Autodesk Fusion 360 part; units mm, degrees
(part 2 of 2)
sketch "Sketch3" plane through (0, -51, 0) normal (0, -1, 0) x (1, 0, 0)
  line L0 (-36, 0) -> (36, 0)
  line L1 (36, 0) -> (36, 24.7)
  line L2 (36, 24.7) -> (-36, 24.7)
  line L3 (-36, 24.7) -> (-36, 0)
  line L4 (-26.5, 21.7) -> (-10.5, 21.7)
  line L5 (-10.5, 21.7) -> (-10.5, 4.7)
  line L6 (-10.5, 4.7) -> (-26.5, 4.7)
  line L7 (-26.5, 4.7) -> (-26.5, 21.7)
  circle A0 centre (16, 11) radius 1.5
  circle A1 centre (25, 13.7) radius 3
  line L8 (-18.5, 21.7) -> (-18.5, 4.7) construction
  line L9 (-26.5, 13.2) -> (-10.5, 13.2) construction
  line L10 (-25, 18.8) -> (-12, 18.8)
  line L11 (-12, 18.8) -> (-12, 7.9)
  line L12 (-12, 7.9) -> (-25, 7.9)
  line L13 (-25, 7.9) -> (-25, 18.8)
  line L14 (-15.25, 7.9) -> (-21.75, 7.9)
  line L15 (-21.75, 7.9) -> (-21.75, 6)
  line L16 (-21.75, 6) -> (-15.25, 6)
  line L17 (-15.25, 6) -> (-15.25, 7.9)
  line L18 (-15.25, 7.9) -> (-21.75, 6) construction
  line L19 (-21.75, 7.9) -> (-15.25, 6) construction
  line L20 (6, 18.8) -> (6, 7.9)
  line L21 (7.5, 21.7) -> (7.5, 4.7)
  line L22 (-7, 7.9) -> (-7, 18.8)
  line L23 (-8.5, 21.7) -> (7.5, 21.7)
  line L24 (-3.75, 7.9) -> (2.75, 6) construction
  line L25 (6, 7.9) -> (-7, 7.9)
  line L26 (-3.75, 7.9) -> (-3.75, 6)
  line L27 (-7, 18.8) -> (6, 18.8)
  line L28 (-8.5, 4.7) -> (-8.5, 21.7)
  line L29 (-8.5, 13.2) -> (7.5, 13.2) construction
  line L30 (-3.75, 6) -> (2.75, 6)
  line L31 (2.75, 6) -> (2.75, 7.9)
  line L32 (2.75, 7.9) -> (-3.75, 6) construction
  line L33 (-0.5, 21.7) -> (-0.5, 4.7) construction
  line L34 (2.75, 7.9) -> (-3.75, 7.9)
  line L35 (7.5, 4.7) -> (-8.5, 4.7)
  circle A2 centre (25, 13.7) radius 0.7
  line L36 (-36, 0) -> (36, 0)
  line L37 (20.725, 18) -> (29.275, 18)
  line L38 (29.275, 18) -> (29.275, 7)
  line L39 (29.275, 7) -> (20.725, 7)
  line L40 (20.725, 7) -> (20.725, 18)
  line L41 (25, 13.7) -> (25, 18) construction
  point P0 (-18.5, 6.95)
  point P1 (-0.5, 6.95)
  dimension "d44" = 16
  dimension "d45" = 17
  dimension "d46" = 1.5
  dimension "d47" = 1.5
  dimension "d48" = 2.9
  dimension "d49" = 3.2
  dimension "d50" = 1.3
  dimension "d51" = 6.5
  dimension "d52" = 9.5
  dimension "d53" = 3
  dimension "d56" = 18
  dimension "d57" = 0
  dimension "d58" = 3
  dimension "d59" = 6
  dimension "d60" = 1.4
  dimension "d61" = 11
  dimension "d62" = 11
  dimension "d63" = 11
  dimension "d64" = 20
  dimension "d67" = 11
  dimension "d68" = 4.3
  dimension "d69" = 8.55
  constraint horizontal L4
  constraint vertical L5
  constraint horizontal L6
  constraint vertical L7
  constraint midpoint L4 L8.start
  constraint midpoint L6 L8.end
  constraint midpoint L7 L9.start
  constraint midpoint L5 L9.end
  constraint horizontal L10
  constraint vertical L11
  constraint horizontal L12
  constraint vertical L13
  constraint horizontal L14
  constraint perpendicular L14 L15
  constraint parallel L14 L16
  constraint parallel L15 L17
  constraint coincident L12 L14.start
  constraint coincident L18 P0
  constraint coincident L19 P0
  constraint coincident L8 P0
  constraint concentric A1 A2
  constraint horizontal L37
  constraint vertical L38
  constraint horizontal L39
  constraint vertical L40
  constraint coincident A1.centre A2.centre
  constraint vertical L41
  constraint symmetric L38 L40 L41
  measures "d44" distance of L5 L7
  measures "d45" distance of L4 L6
  measures "d46" distance of L5 L11
  measures "d47" distance of L7 L13
  measures "d48" distance of L4 L10
  measures "d49" distance of L6 L12
  measures "d50" distance of L6 L16
  measures "d51" distance of L15 L17
  measures "d52" distance of L3 L7
  measures "d53" distance of L2 L4
  measures "d58" diameter of A0
  measures "d59" diameter of A1
  measures "d60" diameter of A2
  measures "d61" distance of L1 A1.centre
  measures "d62" distance of L2 A1.centre
  measures "d63" distance of A0.centre L36
  measures "d64" distance of L1 A0.centre
  measures "d67" distance of L37 L39
  measures "d68" distance of A1.centre L37
  measures "d69" distance of L38 L40
extrude "Extrude5" add sketch "Sketch3" along normal blind 0.3 separate body contours L4 L5 L6 L7 | L21 L23 L28 L35 | L37 L38 L39 L40 makes body 13 at (-2.6667, -51, 20.7333) makes body 14 at (-16.3333, -51, 20.7333) makes body 15 at (24.9253, -51, 8.2361)
extrude "Extrude6" cut sketch "Sketch3" against normal blind 9.6 contours A1 | L10 L11 L12 L13 L14 | L12 L14 L15 L16 L17 | L20 L22 L25 L27 L34 | L25 L26 L30 L31 L34 bodies 1 15 14 13 12 11 10 3 4 9 8 7 6 5 2
extrude "Extrude7" cut sketch "Sketch3" against normal blind 3 contours A0 bodies 11 6 14 13 4 5 10 2 15 3 1 7 12 8 9
sketch "Sketch4" plane through (-36, 0, 0) normal (-1, 0, 0) x (0, -1, 0)
  line L0 (12.6, 1) -> (12.6, 0)
  line L1 (12.6, 0) -> (51, 0)
  line L2 (51, 0) -> (51, 24.7)
  line L3 (51, 24.7) -> (-51, 24.7)
  line L4 (-51, 24.7) -> (-51, 0)
  line L5 (-51, 0) -> (-13.7, 0)
  line L6 (-13.7, 0) -> (-13.7, 1)
  line L7 (-13.7, 1) -> (12.6, 1)
  line L8 (-44, 24.7) -> (-25, 24.7)
  line L9 (-25, 24.7) -> (-25, 0)
  line L10 (-25, 0) -> (-44, 0)
  line L11 (-44, 0) -> (-44, 24.7)
  line L12 (-40.5282, 9.0263) -> (-24.62, 9.0263) construction
  line L13 (-24.62, 9.0263) -> (-24.62, 20.5347) construction
  line L14 (-24.62, 20.5347) -> (-40.5282, 20.5347) construction
  line L15 (-40.5282, 20.5347) -> (-40.5282, 9.0263) construction
  dimension "d74" = 19
  dimension "d75" = 7
  dimension "d78" = 5
  text T0 "SIM" font "Arial" height 5 align left top in box 15.9082 x 11.5083 at (-40.5282, 9.0263) x (1, 0) y (0, 1) spacing 1 kerned
  constraint horizontal L8
  constraint vertical L9
  constraint horizontal L10
  constraint vertical L11
  constraint coincident L3 L8.start
  constraint collinear L5 L10
  measures "d74" distance of L9 L11
  measures "d75" distance of L4 L11
extrude "Extrude8" cut sketch "Sketch4" against normal blind 0.2 contours L3 L5 L8 L9 L10 L11 bodies 9 3 8 13 14 6 7 2 4 1 11 12 10 15 5
extrude "Extrude9" cut sketch "Sketch4" against normal blind 2 text T0 bodies 10 13 1 15 3 12 4 14 9 7 2 8 11 5 6
fillet "Fillet1" radius 1 11 edges at (0, -51, 24.7) (36, 0, 24.7) (36, -51, 12.35) (-36, -13, 24.7) (-36, -51, 12.35) (36, 51, 12.35) (0, 51, 24.7) (-36, 47.5, 24.7) (-35.8, 34.5, 24.7) (-36, 51, 12.35) (-36, 0.55, 1) on bodies 1
equation "d3 = ( 96.2 / 2 ) * 1 mm"
equation "d6 = 16.8 mm - d5"
equation "d7 = 2.45 mm + ( d5 / 2 )"
equation "d9 = 4 mm + d5 / 2"
equation "d11 = 2.2 mm + d10 / 2"
equation "d17 = ( 8 / 2 ) * 1 mm"
equation "d47 = d46"

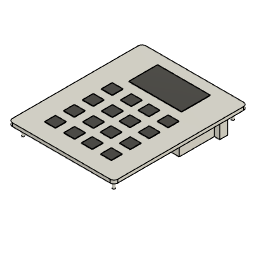
design "CD-100"
Autodesk Fusion 360 part; units mm, degrees
sketch "Cutout" plane through (0, 0, 0) normal (0, 0, 1) x (1, 0, 0)
  line L0 (68.7, -87) -> (-68.7, -87)
  line L1 (-68.7, -87) -> (-68.7, 87)
  line L2 (-68.7, 87) -> (68.7, 87)
  line L3 (68.7, 87) -> (68.7, -87)
  line L4 (68.7, -87) -> (-68.7, 87) construction
  line L5 (-68.7, -87) -> (68.7, 87) construction
  circle A0 centre (-59.055, 77.6351) radius 1.905
  line L6 (0, 0) -> (0, 100) construction
  circle A1 centre (59.055, 77.6351) radius 1.905
  line L7 (0, 0) -> (90, 0) construction
  circle A2 centre (59.055, -77.6351) radius 1.905
  circle A3 centre (-59.055, -77.6351) radius 1.905
  line L8 (-52.9971, 77.6351) -> (52.9971, 77.6351)
  line L9 (52.9971, 77.6351) -> (52.9971, 6.5913)
  line L10 (52.9971, 6.5913) -> (-52.9971, 6.5913)
  line L11 (-52.9971, 6.5913) -> (-52.9971, 77.6351)
  line L12 (-59.055, 72.4281) -> (59.055, 72.4281)
  line L13 (59.055, 72.4281) -> (59.055, 59.7281)
  line L14 (59.055, 59.7281) -> (-59.055, 59.7281)
  line L15 (-59.055, 59.7281) -> (-59.055, 72.4281)
  dimension "d1" = 137.4
  dimension "d2" = 174
  dimension "d7" = 3.81
  dimension "d10" = 118.11
  dimension "d11" = 155.2702
  dimension "d12" = 105.9942
  dimension "d13" = 71.0438
  dimension "d14" = 5.207
  dimension "d15" = 118.11
  dimension "d16" = 12.7
  constraint horizontal L0
  constraint perpendicular L0 L1
  constraint parallel L0 L2
  constraint parallel L1 L3
  constraint coincident L4 L6.start
  constraint coincident L5 L6.start
  constraint coincident L6.start L7.start
  constraint vertical L6
  constraint symmetric A0 L6 A1
  constraint perpendicular L6 L7
  constraint symmetric A0 L7 A3
  constraint symmetric A1 L7 A2
  constraint horizontal L8
  constraint vertical L9
  constraint horizontal L10
  constraint vertical L11
  constraint symmetric L6 L9 L11
  constraint coincident A0.centre L8
  constraint horizontal L12
  constraint vertical L13
  constraint horizontal L14
  constraint vertical L15
  constraint symmetric L6 L13 L15
  measures "d1" distance of L1.end L2.end
  measures "d2" distance of L0.end L1.end
  measures "d7" diameter of A0
  measures "d10" distance of A0.centre A1.centre
  measures "d11" distance of A0.centre A3.centre
  measures "d12" distance of L9 L11
  measures "d13" distance of L8 L10
  measures "d14" distance of A0.centre L12
  measures "d15" distance of L13 L15
  measures "d16" distance of L12 L14
extrude "Extrude1" add sketch "Cutout" along normal blind 4.3 contours L0 L1 L2 L3 | A0 | A1 | A2 | A3 | L8 L9 L11 L12 | L9 L11 L12 L14 | L11 L12 L14 L15 | L9 L12 L13 L14 | L9 L10 L11 L14 makes body 1
sketch "Sketch2" plane through (0, 0, 4.3) normal (0, 0, 1) x (-1, 0, 0)
  line L0 (-68.7, -87) -> (68.7, -87)
  line L1 (68.7, -87) -> (68.7, 87)
  line L2 (68.7, 87) -> (-68.7, 87)
  line L3 (-68.7, 87) -> (-68.7, -87)
sketch "Sketch3" plane through (0, 0, 0) normal (0, 0, -1) x (1, 0, 0)
  line L0 (-68.7, -87) -> (68.7, -87)
  line L1 (68.7, -87) -> (68.7, 87)
  line L2 (68.7, 87) -> (-68.7, 87)
  line L3 (-68.7, 87) -> (-68.7, -87)
  line L4 (-51.9, -14.9) -> (51.9, -14.9)
  line L5 (51.9, -14.9) -> (51.9, -76.4)
  line L6 (51.9, -76.4) -> (-51.9, -76.4)
  line L7 (-51.9, -76.4) -> (-51.9, -14.9)
  line L8 (0, 0) -> (0, 115) construction
  line L9 (-68.7, -87) -> (68.7, -87) construction
  line L10 (58.9, -71.1) -> (-58.9, -71.1)
  line L11 (-58.9, -71.1) -> (-58.9, -60.72)
  line L12 (-58.9, -60.72) -> (58.9, -60.72)
  line L13 (58.9, -60.72) -> (58.9, -71.1)
  circle A0 centre (-59.055, 77.6351) radius 1.65
  circle A1 centre (59.055, 77.6351) radius 1.65
  circle A2 centre (59.055, -77.6351) radius 1.65
  circle A3 centre (-59.055, -77.6351) radius 1.65
  point P0 (-59.055, 77.6351)
  point P1 (59.055, 77.6351)
  point P2 (59.055, -77.6351)
  point P3 (-59.055, -77.6351)
  dimension "d17" = 103.8
  dimension "d18" = 61.5
  dimension "d20" = 10.6
  dimension "d21" = 10.38
  dimension "d22" = 15.9
  dimension "d23" = 7
  dimension "d24" = 7
  dimension "d27" = 3.3
  dimension "d28" = 3.3
  dimension "d29" = 3.3
  dimension "d30" = 3.3
  constraint horizontal L4
  constraint vertical L5
  constraint horizontal L6
  constraint vertical L7
  constraint coincident L8.start origin
  constraint perpendicular L6 L8
  constraint symmetric L5 L7 L8
  constraint horizontal L10
  constraint vertical L11
  constraint horizontal L12
  constraint vertical L13
  constraint coincident P0 A0.centre
  constraint coincident P1 A1.centre
  constraint coincident P2 A2.centre
  constraint coincident P3 A3.centre
  measures "d17" distance of L5 L7
  measures "d18" distance of L4 L6
  measures "d20" distance of L6 L9
  measures "d21" distance of L10 L12
  measures "d22" distance of L9 L10
  measures "d23" distance of L7 L11
  measures "d24" distance of L5 L13
  measures "d27" diameter of A0
  measures "d28" diameter of A1
  measures "d29" diameter of A2
  measures "d30" diameter of A3
extrude "Extrude2" add sketch "Sketch3" along normal blind 27.3 contours L4 L5 L7 L12 | L5 L7 L10 L12 | L7 L10 L11 L12 | L5 L10 L12 L13 | L5 L6 L7 L10 bodies 1
extrude "Extrude3" add sketch "Sketch3" along normal blind 12.7 separate body contours A0 | A1 | A2 | A3 makes body 2 at (60.4629, -78.4955, -8.4667) makes body 3 at (60.4629, 76.7747, -8.4667) makes body 4 at (-57.6471, -78.4955, -8.4667) makes body 5 at (-57.6471, 76.7747, -8.4667)
sketch "Sketch4" plane through (0, 0, -27.3) normal (0, 0, -1) x (1, 0, 0)
  line L0 (58.9, -60.72) -> (51.9, -60.72)
  line L1 (51.9, -60.72) -> (51.9, -14.9)
  line L2 (51.9, -14.9) -> (-51.9, -14.9)
  line L3 (-51.9, -14.9) -> (-51.9, -60.72)
  line L4 (-51.9, -60.72) -> (-58.9, -60.72)
  line L5 (-58.9, -60.72) -> (-58.9, -71.1)
  line L6 (-58.9, -71.1) -> (-51.9, -71.1)
  line L7 (-51.9, -71.1) -> (-51.9, -76.4)
  line L8 (-51.9, -76.4) -> (51.9, -76.4)
  line L9 (51.9, -76.4) -> (51.9, -71.1)
  line L10 (51.9, -71.1) -> (58.9, -71.1)
  line L11 (58.9, -71.1) -> (58.9, -60.72)
  line L12 (8.9, -34.92) -> (-8.9, -34.92)
  line L13 (-8.9, -34.92) -> (-8.9, -25.6)
  line L14 (-8.9, -25.6) -> (8.9, -25.6)
  line L15 (8.9, -25.6) -> (8.9, -34.92)
  line L16 (8.9, -34.92) -> (7, -25.6)
  line L17 (-8.9, -34.92) -> (-7, -25.6)
  line L18 (0, 0) -> (0, -100)
  line L19 (-51.9, -14.9) -> (51.9, -14.9)
  dimension "d33" = 17.8
  dimension "d34" = 9.32
  dimension "d35" = 10.7
  dimension "d36" = 14
  constraint horizontal L12
  constraint vertical L13
  constraint horizontal L14
  constraint vertical L15
  constraint coincident L14 L16.end
  constraint coincident L14 L17.end
  constraint symmetric L13 L15 L18
  constraint symmetric L16 L17 L18
  measures "d33" distance of L13 L15
  measures "d34" distance of L12 L14
  measures "d35" distance of L14 L19
  measures "d36" distance of L16.end L17.end
extrude "Extrude4" add sketch "Sketch4" along normal blind 4 separate body contours L12 L14 L17 L18 | L12 L14 L16 L18 makes body 6
fillet "Fillet1" radius 5 4 edges at (68.7, 87, 2.15) (-68.7, 87, 2.15) (68.7, -87, 2.15) (-68.7, -87, 2.15) on bodies 1
sketch "Sketch5" plane through (0, 0, 4.3) normal (0, 0, 1) x (-1, 0, 0)
  arc A0 (68.7, 82) -> (63.7, 87) centre (63.7, 82) ccw
  line L0 (63.7, 87) -> (-63.7, 87)
  arc A1 (-63.7, 87) -> (-68.7, 82) centre (-63.7, 82) ccw
  line L1 (-68.7, 82) -> (-68.7, -82)
  arc A2 (-68.7, -82) -> (-63.7, -87) centre (-63.7, -82) ccw
  line L2 (-63.7, -87) -> (63.7, -87)
  arc A3 (63.7, -87) -> (68.7, -82) centre (63.7, -82) ccw
  line L3 (68.7, -82) -> (68.7, 82)
  line L4 (34.1972, -72.7537) -> (-34.5148, -72.7537)
  line L5 (-34.5148, -72.7537) -> (-34.5148, -35.3411)
  line L6 (-34.5148, -35.3411) -> (34.1972, -35.3411)
  line L7 (34.1972, -35.3411) -> (34.1972, -72.7537)
  line L8 (43.5437, -22.886) -> (29.4463, -22.886)
  line L9 (29.4463, -22.886) -> (29.4463, -8.7887)
  line L10 (29.4463, -8.7887) -> (43.5437, -8.7887)
  line L11 (43.5437, -8.7887) -> (43.5437, -22.886)
  line L12 (0, 0) -> (0, -100) construction
  line L13 (4.4463, -8.7887) -> (18.5437, -8.7887)
  line L14 (18.5437, -8.7887) -> (18.5437, -22.886)
  line L15 (18.5437, -22.886) -> (4.4463, -22.886)
  line L16 (4.4463, -22.886) -> (4.4463, -8.7887)
  line L17 (-4.4463, -22.886) -> (-4.4463, -8.7887)
  line L18 (-4.4463, -8.7887) -> (-18.5437, -8.7887)
  line L19 (-43.5437, -8.7887) -> (-43.5437, -22.886)
  line L20 (-18.5437, -22.886) -> (-4.4463, -22.886)
  line L21 (-29.4463, -8.7887) -> (-43.5437, -8.7887)
  line L22 (-18.5437, -8.7887) -> (-18.5437, -22.886)
  line L23 (-29.4463, -22.886) -> (-29.4463, -8.7887)
  line L24 (-43.5437, -22.886) -> (-29.4463, -22.886)
  line L25 (-43.5437, 1.7806) -> (-29.4463, 1.7806)
  line L26 (-4.4463, 1.7806) -> (-4.4463, 15.878)
  line L27 (-29.4463, 1.7806) -> (-29.4463, 15.878)
  line L28 (29.4463, 1.7806) -> (29.4463, 15.878)
  line L29 (29.4463, 15.878) -> (43.5437, 15.878)
  line L30 (-43.5437, 15.878) -> (-43.5437, 1.7806)
  line L31 (4.4463, 1.7806) -> (4.4463, 15.878)
  line L32 (4.4463, 15.878) -> (18.5437, 15.878)
  line L33 (-29.4463, 15.878) -> (-43.5437, 15.878)
  line L34 (-4.4463, 15.878) -> (-18.5437, 15.878)
  line L35 (43.5437, 15.878) -> (43.5437, 1.7806)
  line L36 (43.5437, 1.7806) -> (29.4463, 1.7806)
  line L37 (18.5437, 1.7806) -> (4.4463, 1.7806)
  line L38 (-18.5437, 1.7806) -> (-4.4463, 1.7806)
  line L39 (-18.5437, 15.878) -> (-18.5437, 1.7806)
  line L40 (18.5437, 15.878) -> (18.5437, 1.7806)
  line L41 (-43.5437, 26.4473) -> (-29.4463, 26.4473)
  line L42 (-4.4463, 26.4473) -> (-4.4463, 40.5447)
  line L43 (-29.4463, 26.4473) -> (-29.4463, 40.5447)
  line L44 (29.4463, 26.4473) -> (29.4463, 40.5447)
  line L45 (29.4463, 40.5447) -> (43.5437, 40.5447)
  line L46 (-43.5437, 40.5447) -> (-43.5437, 26.4473)
  line L47 (4.4463, 26.4473) -> (4.4463, 40.5447)
  line L48 (4.4463, 40.5447) -> (18.5437, 40.5447)
  line L49 (-29.4463, 40.5447) -> (-43.5437, 40.5447)
  line L50 (-4.4463, 40.5447) -> (-18.5437, 40.5447)
  line L51 (43.5437, 40.5447) -> (43.5437, 26.4473)
  line L52 (43.5437, 26.4473) -> (29.4463, 26.4473)
  line L53 (18.5437, 26.4473) -> (4.4463, 26.4473)
  line L54 (-18.5437, 26.4473) -> (-4.4463, 26.4473)
  line L55 (-18.5437, 40.5447) -> (-18.5437, 26.4473)
  line L56 (18.5437, 40.5447) -> (18.5437, 26.4473)
  line L57 (-43.5437, 51.114) -> (-29.4463, 51.114)
  line L58 (-4.4463, 51.114) -> (-4.4463, 65.2113)
  line L59 (-29.4463, 51.114) -> (-29.4463, 65.2113)
  line L60 (29.4463, 51.114) -> (29.4463, 65.2113)
  line L61 (29.4463, 65.2113) -> (43.5437, 65.2113)
  line L62 (-43.5437, 65.2113) -> (-43.5437, 51.114)
  line L63 (4.4463, 51.114) -> (4.4463, 65.2113)
  line L64 (4.4463, 65.2113) -> (18.5437, 65.2113)
  line L65 (-29.4463, 65.2113) -> (-43.5437, 65.2113)
  line L66 (-4.4463, 65.2113) -> (-18.5437, 65.2113)
  line L67 (43.5437, 65.2113) -> (43.5437, 51.114)
  line L68 (43.5437, 51.114) -> (29.4463, 51.114)
  line L69 (18.5437, 51.114) -> (4.4463, 51.114)
  line L70 (-18.5437, 51.114) -> (-4.4463, 51.114)
  line L71 (-18.5437, 65.2113) -> (-18.5437, 51.114)
  line L72 (18.5437, 65.2113) -> (18.5437, 51.114)
  dimension "d43" = 0
  dimension "d44" = 74
  constraint horizontal L4
  constraint vertical L5
  constraint horizontal L6
  constraint vertical L7
  constraint horizontal L8
  constraint vertical L9
  constraint horizontal L10
  constraint vertical L11
  constraint coincident L12.start origin
  constraint perpendicular L6 L12
  constraint horizontal L15
  constraint vertical L16
  constraint horizontal L13
  constraint vertical L14
  constraint symmetric L8.start L12 L19.end
  constraint symmetric L8.end L12 L23.start
  constraint symmetric L9.end L12 L21.start
  constraint symmetric L10.end L12 L19.start
  constraint symmetric L12 L15.end L17.start
  constraint symmetric L12 L14.end L20.start
  constraint symmetric L12 L13.end L18.end
  constraint symmetric L12 L13.start L17.end
extrude "Extrude5" add sketch "Sketch5" along normal blind 0.6 separate body contours L4 L5 L6 L7 | L8 L9 L10 L11 | L13 L14 L15 L16 | L17 L18 L20 L22 | L19 L21 L23 L24 | L25 L27 L30 L33 | L26 L34 L38 L39 | L28 L29 L35 L36 | L31 L32 L37 L40 | L41 L43 L46 L49 | L42 L50 L54 L55 | L44 L45 L51 L52 | L47 L48 L53 L56 | L57 L59 L62 L65 | L58 L66 L70 L71 | L60 L61 L67 L68 | L63 L64 L69 L72 makes body 7 at (9.1455, -55.8131, 4.3) makes body 8 at (-9.1455, -35.8455, 4.3) makes body 9 at (9.1455, -6.4797, 4.3) makes body 10 at (-9.1455, 18.1869, 4.3) makes body 11 at (-38.8446, 18.1869, 4.3) makes body 12 at (38.8446, -11.1789, 4.3) makes body 13 at (-34.1455, -31.1464, 4.3) makes body 14 at (38.8446, -60.5122, 4.3) makes body 15 at (-9.1455, -55.8131, 4.3) makes body 16 at (13.8446, -31.1464, 4.3) makes body 17 at (-9.1455, -11.1789, 4.3) makes body 18 at (38.8446, 13.4878, 4.3) makes body 19 at (11.6108, 47.812, 4.3) makes body 20 at (9.1455, 18.1869, 4.3) makes body 21 at (-34.1455, -6.4797, 4.3) makes body 22 at (38.8446, -31.1464, 4.3) makes body 23 at (-34.1455, -60.5122, 4.3)
equation "d12 = ( 4.412 in - 0.239 in )"
equation "d16 = 0.705 in - d14"
equation "d24 = d23"
equation "d28 = d27"
equation "d29 = d28"
equation "d30 = d29"
